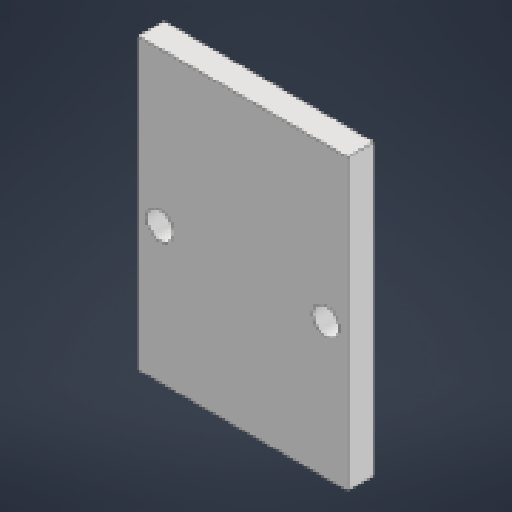
# Autodesk Inventor part: 触点外壳
Saved by Autodesk Inventor 2025 (Build 290162000, 162)
## iProperties
Created: 2026-04-17
Part Number: 触点外壳
Material: 常规
Document SubType Name: Modeling
Designer: XH
Density: 1 g/cm^3
Appearance: 默认
Author: XH
Autodesk Inventor part; units mm, degrees
ref_plane "YZ Plane" through (0, 0, 0) normal (1, 0, 0) x (0, 1, 0)
ref_plane "XZ Plane" through (0, 0, 0) normal (0, 1, 0) x (-1, 0, 0)
ref_plane "XY Plane" through (0, 0, 0) normal (0, 0, 1) x (1, 0, 0)
sketch "草图1" plane through (0, 0, 0) normal (0, 0, 1) x (1, 0, 0)
  circle A0 centre (-9.405, -0.7961) radius 2 projected
  line L0 (-4.9391, -16.3471) -> (-4.9391, -13.3471) projected
  line L1 (-4.9391, -13.3471) -> (-6.4391, -13.3471) projected
  line L2 (-6.4391, -13.3471) -> (-6.4391, 13.6529) projected
  line L3 (-4.9391, 13.6529) -> (-6.4391, 13.6529) projected
  line L4 (-4.9391, 16.6529) -> (-4.9391, 13.6529) projected
  line L5 (-4.9391, 16.6529) -> (-11.9051, 16.6529) projected
  line L6 (-11.9051, 16.6529) -> (-11.9051, -16.3471) projected
  line L7 (-4.9391, -16.3471) -> (-11.9051, -16.3471) projected
  circle A1 centre (9.5269, -0.7961) radius 2 projected
  line L8 (5.0609, -16.3471) -> (12.0269, -16.3471) projected
  line L9 (12.0269, -16.3471) -> (12.0269, 16.6529) projected
  line L10 (5.0609, 16.6529) -> (12.0269, 16.6529) projected
  line L11 (5.0609, 16.6529) -> (5.0609, 13.6529) projected
  line L12 (6.5609, 13.6529) -> (5.0609, 13.6529) projected
  line L13 (6.5609, -13.3471) -> (6.5609, 13.6529) projected
  line L14 (6.5609, -13.3471) -> (5.0609, -13.3471) projected
  line L15 (5.0609, -13.3471) -> (5.0609, -16.3471) projected
  line L16 (12.0269, -16.3471) -> (-11.9051, -16.3471)
  line L17 (-11.9051, -16.3471) -> (-11.9051, 16.6529)
  line L18 (-11.9051, 16.6529) -> (12.0269, 16.6529)
  line L19 (12.0269, 16.6529) -> (12.0269, -16.3471)
  circle A2 centre (9.5269, -0.7961) radius 1.5
  circle A3 centre (-9.405, -0.7961) radius 1.5
  dimension "d2" = 0.5
  dimension "d3" = 0.5
  constraints: 8 end point, 2 centre point, 2 parallel, 1 horizontal, 1 perpendicular
  measures "d2" radial gap between concentric circles of A1 A2
  measures "d3" radial gap between concentric circles of A0 A3
extrude "拉伸1" add sketch "草图1" along normal blind 3 contours A0 | L7 L6 L5 L4 L3 L2 L1 L0 | L0 L1 L2 L3 L4 L18 L11 L12 L13 L14 L15 L16 | L15 L14 L13 L12 L11 L10 L9 L8 | A1
